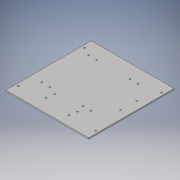
# Autodesk Inventor part: BottomPlate
Saved by Autodesk Inventor 2016 (Build 200138000, 138)
## iProperties
Created: 2015-08-28
Part Number: BottomPlate
Material: Generic
Document SubType Name: Modeling
Designer: lachesis
Density: 1 g/cm^3
Appearance: Default
Author: lachesis
Autodesk Inventor part; units mm, degrees
ref_plane "YZ Plane" through (0, 0, 0) normal (1, 0, 0) x (0, 1, 0)
ref_plane "XZ Plane" through (0, 0, 0) normal (0, 1, 0) x (-1, 0, 0)
ref_plane "XY Plane" through (0, 0, 0) normal (0, 0, 1) x (1, 0, 0)
sketch "Block1" plane through (0, 0, 0) normal (0, 0, 1) x (1, 0, 0)
  circle A0 centre (244.9891, 313.0766) radius 1.651
  circle A1 centre (305.4278, 286.7035) radius 1.651
  circle A2 centre (242.5353, 295.4667) radius 1.651
  circle A3 centre (307.8815, 304.3134) radius 1.651
  circle A4 centre (325.7478, 277.8135) radius 1.651
  circle A5 centre (227.9578, 277.8135) radius 1.651
  circle A6 centre (194.5568, 203.1375) radius 1.651
  circle A7 centre (325.7478, 166.5615) radius 1.651
  circle A8 centre (227.9578, 166.5615) radius 1.651
  circle A9 centre (247.0078, 166.5615) radius 1.651
  circle A10 centre (344.7978, 166.5615) radius 1.651
  circle A11 centre (194.5568, 241.2375) radius 1.651
  circle A12 centre (247.0078, 277.8135) radius 1.651
  circle A13 centre (344.7978, 277.8135) radius 1.651
  circle A14 centre (181.8568, 156.6555) radius 1.905
  circle A15 centre (181.8568, 312.8401) radius 1.905
  circle A16 centre (365.194, 312.8401) radius 1.905
  circle A17 centre (365.194, 156.6555) radius 1.905
  line L0 (371.544, 133.5415) -> (371.544, 335.9541)
  line L1 (175.5068, 133.5415) -> (371.544, 133.5415)
  line L2 (175.5068, 335.9541) -> (175.5068, 133.5415)
  line L3 (371.544, 335.9541) -> (175.5068, 335.9541)
  point P0 (271.6644, 239.9388)
sketch "Sketch1" plane through (0, 0, 0) normal (0, 1, 0) x (-1, 0, 0)
  circle A0 centre (-28.5363, 78.3288) radius 1.651
  circle A1 centre (31.9024, 51.9557) radius 1.651
  circle A2 centre (-30.99, 60.7189) radius 1.651
  circle A3 centre (34.3561, 69.5656) radius 1.651
  circle A4 centre (52.2224, 43.0657) radius 1.651
  circle A5 centre (-45.5676, 43.0657) radius 1.651
  circle A6 centre (-78.9686, -31.6103) radius 1.651
  circle A7 centre (52.2224, -68.1863) radius 1.651
  circle A8 centre (-45.5676, -68.1863) radius 1.651
  circle A9 centre (-26.5176, -68.1863) radius 1.651
  circle A10 centre (71.2724, -68.1863) radius 1.651
  circle A11 centre (-78.9686, 6.4897) radius 1.651
  circle A12 centre (-26.5176, 43.0657) radius 1.651
  circle A13 centre (71.2724, 43.0657) radius 1.651
  circle A14 centre (-91.6686, -78.0923) radius 1.905
  circle A15 centre (-91.6686, 78.0923) radius 1.905
  circle A16 centre (91.6686, 78.0923) radius 1.905
  circle A17 centre (91.6686, -78.0923) radius 1.905
  line L0 (98.0186, -101.2063) -> (98.0186, 101.2063)
  line L1 (-98.0186, -101.2063) -> (98.0186, -101.2063)
  line L2 (-98.0186, 101.2063) -> (-98.0186, -101.2063)
  line L3 (98.0186, 101.2063) -> (-98.0186, 101.2063)
  point P0 (0, 0)
  point P1 (0, -101.2063)
  point P2 (-98.0186, 0)
  constraints: 1 horizontal alignment, 1 vertical alignment, 2 other
extrude "Extrusion1" add sketch "Sketch1" along normal blind 3
body "Solid1"
